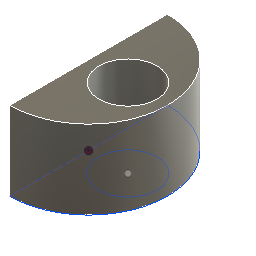
Holder (Autodesk Fusion 360 design; units mm, degrees)
Autodesk Fusion 360 part; units mm, degrees
sketch "Sketch1" plane through (0, 0, 0) normal (0, 1, 0) x (1, 0, 0)
  arc A0 (0, -15) -> (0, 15) centre (0, 0) ccw
  line L0 (0, 0) -> (0, -15) construction
  line L1 (0, 0) -> (0, 15) construction
  line L2 (0, 15) -> (0, -15)
  circle A1 centre (7.5, 0) radius 5.5
  dimension "d1" = 180
  dimension "d2" = 11
  dimension "d10" = 7.5
  measures "d1" angle of L0 L1
  measures "d2" diameter of A1
  measures "d10" distance of L2
extrude "Extrude1" add sketch "Sketch1" along normal blind 15
extrude "Extrude2" add sketch "Sketch1" along normal blind 25 contours A1
extrude "Extrude3" cut 1 faces at (7.6099, 25, -1.4661) along direction (0, -1, 0) blind 30
